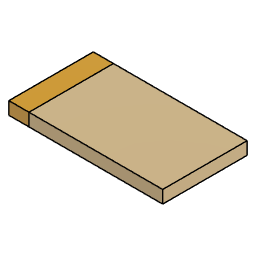
ProjectDesign (Autodesk Fusion 360 archive; units mm, degrees)
design "Battery"
Autodesk Fusion 360 part; units mm, degrees
sketch "Sketch8" plane through (0, 0, 6.3) normal (0, 0, 1) x (-1, 0, 0)
sketch "Sketch10" plane through (0, 0, 6.3) normal (0, 0, 1) x (-1, 0, 0)
sketch "Sketch11" plane through (0, 0, 0) normal (0, -1, 0) x (1, 0, 0)
sketch "Sketch12" plane through (0, 0, 0) normal (0, 0, -1) x (1, 0, 0)
sketch "Sketch13" plane through (0, 42, 0) normal (0, 1, 0) x (-1, 0, 0)
box "BoxPrimitive9" add length 42 width 66.5 height 6.3 placed x (0, 1, 0) y (-1, 0, 0) z (0, 0, 1) at (66.5, 0, 0) makes body 1
box "BoxPrimitive10" add length 42 width 10 height -6.3 placed x (0, -1, 0) y (1, 0, 0) z (0, 0, 1) at (-10, 42, 6.3) separate body makes body 2
copy_body "Body->Comp1" bodies 2 removing the originals makes body 3 in component "Component'"
copy_body "Body->Comp2" bodies 1 removing the originals makes body 4 in component "Component''"
component "Component" placed x (1, 0, 0) y (0, 1, 0) z (0, 0, 1) at (0, 0, 0)
component "Component'" placed x (1, 0, 0) y (0, 1, 0) z (0, 0, 1) at (0, 0, 0)
component "Component''" placed x (1, 0, 0) y (0, 1, 0) z (0, 0, 1) at (0, 0, 0)

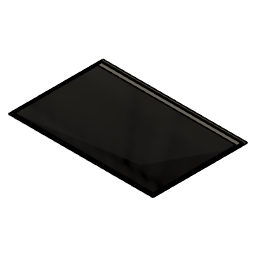
design "Display"
Autodesk Fusion 360 part; units mm, degrees
box "BoxPrimitive1" add length 111.2 width 170.2 height 0.48 placed x (0, 1, 0) y (-1, 0, 0) z (0, 0, 1) at (170.2, 0, 0) makes body 1
box "BoxPrimitive2" add length 107.09 width 167.8 height 0.23 placed x (0, 1, 0) y (-1, 0, 0) z (0, 0, 1) at (167.8, 0, 0.48) separate body makes body 2
move_body "Move1" bodies 2 to x (1, 0, 0) y (0, 1, 0) z (0, 0, 1) at (1.2, 1.2, 0)
box "BoxPrimitive3" add length 104.09 width 164.8 height 0.23 placed x (0, 1, 0) y (-1, 0, 0) z (0, 0, 1) at (166, 1.2, 0.71) separate body makes body 3
move_body "Move2" bodies 3 to x (1, 0, 0) y (0, 1, 0) z (0, 0, 1) at (1.5, 1.5, 0)
box "BoxPrimitive4" add length 97.92 width 163.2 height 0.23 placed x (0, 1, 0) y (-1, 0, 0) z (0, 0, 1) at (165.9, 2.7, 0.94) separate body makes body 4
move_body "Move3" bodies 4 to x (1, 0, 0) y (0, 1, 0) z (0, 0, 1) at (0.8, 0.8, 0)
copy_body "Body->Comp1" bodies 4 removing the originals makes body 5 in component "Component"
copy_body "Body->Comp2" bodies 3 removing the originals makes body 6 in component "Component'"
copy_body "Body->Comp3" bodies 2 removing the originals makes body 7 in component "Component''"
copy_body "Body->Comp4" bodies 1 removing the originals makes body 8 in component "Component'''"
component "Component" placed x (1, 0, 0) y (0, 1, 0) z (0, 0, 1) at (0, 0, 0)
component "Component'" placed x (1, 0, 0) y (0, 1, 0) z (0, 0, 1) at (0, 0, 0)
component "Component''" placed x (1, 0, 0) y (0, 1, 0) z (0, 0, 1) at (0, 0, 0)
component "Component'''" placed x (1, 0, 0) y (0, 1, 0) z (0, 0, 1) at (0, 0, 0)
